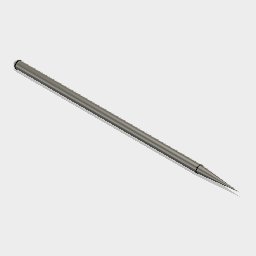
铅笔 (Autodesk Fusion 360 design; units mm, degrees)
Autodesk Fusion 360 part; units mm, degrees
cylinder "圆柱体基本要素1" add diameter 4 height 100 placed x (0, 0, -1) y (0, 1, 0) z (1, 0, 0) at (0, 0, 0) makes body 1
sphere "球体基本要素1" add diameter 4 placed x (1, 0, 0) y (0, 1, 0) z (0, 0, 1) at (13.2511, 25.9041, 0) separate body makes body 2
move_body "对齐1" bodies 2 to x (1, 0, 0) y (0, 1, 0) z (0, 0, 1) at (-13.2511, -25.9041, -2)
move_body "对齐2" bodies 2 to x (0, 0, 1) y (0, 1, 0) z (-1, 0, 0) at (-2, 0, 0)
sketch "草图3" plane through (0, 0, 0) normal (0, 0, 1) x (1, 0, 0)
extrude "拉伸1" add 1 faces at (100, 0.1965, -0.637) along direction (1, 0, 0) blind 23 draft -5 on bodies 1 bodies 1
